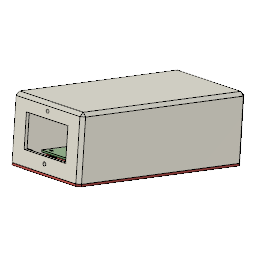
c64-psu-2018.2 v1 (Autodesk Fusion 360 design; units mm, degrees)
Autodesk Fusion 360 part; units mm, degrees
note: some values were not read from the file. Chosen so that the rebuilt part matches the saved one: which face or edge a step refers to; which pieces of a blend or face edit are solid.
sketch "PCB" plane through (0, 0, 0) normal (0, 0, 1) x (1, 0, 0)
  line L0 (0, 0) -> (117, 0)
  line L1 (117, 0) -> (117, 74)
  line L2 (117, 74) -> (0, 74)
  line L3 (0, 74) -> (0, 0)
  circle A0 centre (5, 69) radius 1.6
  circle A1 centre (5, 5) radius 1.6
  circle A2 centre (112, 69) radius 1.6
  circle A3 centre (112, 5) radius 1.6
  dimension "d1" = 74
  dimension "d2" = 117
  dimension "d5" = 3.2
  dimension "d6" = 5
  dimension "d7" = 5
  dimension "d10" = 3.2
  dimension "d11" = 5
  dimension "d12" = 5
  dimension "d13" = 3.2
  dimension "d14" = 3.2
  dimension "d15" = 5
  dimension "d16" = 5
  dimension "d17" = 5
  dimension "d18" = 5
  measures "d5" diameter of A0
  measures "d6" distance of L0.start
  measures "d7" distance of L0.start
  measures "d10" diameter of A1
  measures "d13" diameter of A2
  measures "d14" diameter of A3
extrude "Extrude6" add sketch "PCB" along normal blind 1.6 makes body 1
move_body "Move1" bodies 1 to x (1, 0, 0) y (0, 1, 0) z (0, 0, 1) at (0, 0, 7)
sketch "bottom sketch" plane through (0, 0, 0) normal (0, 0, 1) x (1, 0, 0)
  line L0 (-28, 77) -> (129, 77)
  line L1 (129, 77) -> (129, -3)
  line L2 (129, -3) -> (-28, -3)
  line L3 (-28, -3) -> (-28, 77)
  line L4 (126.2, -0.2) -> (-25.2, -0.2)
  line L5 (-25.2, -0.2) -> (-25.2, 74.2)
  line L6 (-25.2, 74.2) -> (126.2, 74.2)
  line L7 (126.2, 74.2) -> (126.2, -0.2)
  line L8 (-25.2, 74.2) -> (-16.2, 74.2)
  line L9 (-16.2, 74.2) -> (-16.2, 65.2)
  line L10 (-16.2, 65.2) -> (-25.2, 65.2)
  line L11 (-25.2, 65.2) -> (-25.2, 74.2)
  line L12 (-25.2, -0.2) -> (-16.2, -0.2)
  line L13 (-16.2, -0.2) -> (-16.2, 8.8)
  line L14 (-16.2, 8.8) -> (-25.2, 8.8)
  line L15 (-25.2, 8.8) -> (-25.2, -0.2)
  line L16 (126.2, -0.2) -> (117.2, -0.2)
  line L17 (117.2, -0.2) -> (117.2, 8.8)
  line L18 (117.2, 8.8) -> (126.2, 8.8)
  line L19 (126.2, 8.8) -> (126.2, -0.2)
  line L20 (126.2, 74.2) -> (117.2, 74.2)
  line L21 (117.2, 74.2) -> (117.2, 65.2)
  line L22 (117.2, 65.2) -> (126.2, 65.2)
  line L23 (126.2, 65.2) -> (126.2, 74.2)
  line L24 (-17.55, 69.7) -> (-19.125, 72.428)
  line L25 (-19.125, 72.428) -> (-22.275, 72.428)
  line L26 (-22.275, 72.428) -> (-23.85, 69.7)
  line L27 (-23.85, 69.7) -> (-22.275, 66.972)
  line L28 (-22.275, 66.972) -> (-19.125, 66.972)
  line L29 (-19.125, 66.972) -> (-17.55, 69.7)
  line L30 (-17.55, 4.3) -> (-19.125, 7.028)
  line L31 (-19.125, 7.028) -> (-22.275, 7.028)
  line L32 (-22.275, 7.028) -> (-23.85, 4.3)
  line L33 (-23.85, 4.3) -> (-22.275, 1.572)
  line L34 (-22.275, 1.572) -> (-19.125, 1.572)
  line L35 (-19.125, 1.572) -> (-17.55, 4.3)
  line L36 (124.85, 69.7) -> (123.275, 72.428)
  line L37 (123.275, 72.428) -> (120.125, 72.428)
  line L38 (120.125, 72.428) -> (118.55, 69.7)
  line L39 (118.55, 69.7) -> (120.125, 66.972)
  line L40 (120.125, 66.972) -> (123.275, 66.972)
  line L41 (123.275, 66.972) -> (124.85, 69.7)
  line L42 (124.85, 4.3) -> (123.275, 7.028)
  line L43 (123.275, 7.028) -> (120.125, 7.028)
  line L44 (120.125, 7.028) -> (118.55, 4.3)
  line L45 (118.55, 4.3) -> (120.125, 1.572)
  line L46 (120.125, 1.572) -> (123.275, 1.572)
  line L47 (123.275, 1.572) -> (124.85, 4.3)
  circle A0 centre (-20.7, 69.7) radius 1.6
  circle A1 centre (-20.7, 4.3) radius 1.6
  circle A2 centre (121.7, 4.3) radius 1.6
  circle A3 centre (121.7, 69.7) radius 1.6
  circle A4 centre (5, 69) radius 4
  circle A5 centre (112, 69) radius 4
  circle A6 centre (5, 5) radius 4
  circle A7 centre (112, 5) radius 4
  dimension "d22" = 3
  dimension "d23" = 3
  dimension "d24" = 28
  dimension "d25" = 12
  dimension "d60" = 2.8
  dimension "d61" = 9
  dimension "d62" = 9
  dimension "d63" = 9
  dimension "d64" = 9
  dimension "d65" = 9
  dimension "d66" = 9
  dimension "d67" = 9
  dimension "d68" = 9
  dimension "d69" = 3.15
  dimension "d70" = 4.5
  dimension "d71" = 4.5
  dimension "d72" = 3.15
  dimension "d73" = 4.5
  dimension "d74" = 4.5
  dimension "d75" = 3.15
  dimension "d76" = 4.5
  dimension "d77" = 4.5
  dimension "d78" = 3.15
  dimension "d79" = 4.5
  dimension "d80" = 4.5
  dimension "d81" = 3.2
  dimension "d82" = 3.2
  dimension "d83" = 3.2
  dimension "d84" = 3.2
  dimension "d111" = 8
  dimension "d112" = 8
  dimension "d113" = 8
  dimension "d114" = 8
  measures "d22" distance of origin
  measures "d60" distance of L2
  measures "d61" distance of origin
  measures "d63" distance of origin
  measures "d64" distance of origin
  measures "d66" distance of origin
  measures "d69" distance of origin
  measures "d73" distance of origin
  measures "d74" distance of origin
  measures "d79" distance of origin
  measures "d80" distance of origin
  measures "d81" diameter of A0
  measures "d82" diameter of A1
  measures "d83" diameter of A2
  measures "d84" diameter of A3
  measures "d111" diameter of A4
  measures "d112" diameter of A5
  measures "d113" diameter of A6
  measures "d114" diameter of A7
sketch "bounding box" plane through (0, 0, 0) normal (0, 0, 1) x (1, 0, 0)
  line L0 (-28, 77) -> (129, 77)
  line L1 (129, 77) -> (129, -3)
  line L2 (129, -3) -> (-28, -3)
  line L3 (-28, -3) -> (-28, 77)
sketch "bottom bolt recess" plane through (0, 0, 0) normal (0, 0, 1) x (1, 0, 0)
  circle A0 centre (-20.7, 69.7) radius 2.85
  circle A1 centre (-20.7, 4.3) radius 2.85
  circle A2 centre (121.7, 69.7) radius 2.85
  circle A3 centre (121.7, 4.3) radius 2.85
  dimension "d105" = 5.7
  dimension "d106" = 5.7
  dimension "d107" = 5.7
  dimension "d108" = 5.7
  measures "d105" diameter of A0
  measures "d106" diameter of A1
  measures "d107" diameter of A2
  measures "d108" diameter of A3
sketch "PCB nut recess" plane through (0, 0, 0) normal (0, 0, 1) x (1, 0, 0)
  line L0 (6.575, 66.272) -> (8.15, 69)
  line L1 (8.15, 69) -> (6.575, 71.728)
  line L2 (6.575, 71.728) -> (3.425, 71.728)
  line L3 (3.425, 71.728) -> (1.85, 69)
  line L4 (1.85, 69) -> (3.425, 66.272)
  line L5 (3.425, 66.272) -> (6.575, 66.272)
  line L6 (8.15, 5) -> (6.575, 7.728)
  line L7 (6.575, 7.728) -> (3.425, 7.728)
  line L8 (3.425, 7.728) -> (1.85, 5)
  line L9 (1.85, 5) -> (3.425, 2.272)
  line L10 (3.425, 2.272) -> (6.575, 2.272)
  line L11 (6.575, 2.272) -> (8.15, 5)
  line L12 (110.425, 66.272) -> (113.575, 66.272)
  line L13 (113.575, 66.272) -> (115.15, 69)
  line L14 (115.15, 69) -> (113.575, 71.728)
  line L15 (113.575, 71.728) -> (110.425, 71.728)
  line L16 (110.425, 71.728) -> (108.85, 69)
  line L17 (108.85, 69) -> (110.425, 66.272)
  line L18 (108.3627, 5) -> (110.1813, 1.85)
  line L19 (110.1813, 1.85) -> (113.8187, 1.85)
  line L20 (113.8187, 1.85) -> (115.6373, 5)
  line L21 (115.6373, 5) -> (113.8187, 8.15)
  line L22 (113.8187, 8.15) -> (110.1813, 8.15)
  line L23 (110.1813, 8.15) -> (108.3627, 5)
  dimension "d118" = 3.15
  dimension "d119" = 3.15
  dimension "d120" = 3.15
  dimension "d121" = 3.15
  measures "d121" distance of L23
sketch "PCB holes" plane through (0, 0, 0) normal (0, 0, 1) x (1, 0, 0)
  circle A0 centre (5, 69) radius 1.6
  circle A1 centre (5, 5) radius 1.6
  circle A2 centre (112, 69) radius 1.6
  circle A3 centre (112, 5) radius 1.6
  dimension "d124" = 3.2
  dimension "d125" = 3.2
  dimension "d126" = 3.2
  dimension "d127" = 3.2
  measures "d124" diameter of A0
  measures "d125" diameter of A1
  measures "d126" diameter of A2
  measures "d127" diameter of A3
extrude "Extrude9" add sketch "bottom sketch" along normal blind 2 separate body contours L0 L1 L2 L3 makes body 2
extrude "Extrude10" add sketch "bottom sketch" along normal blind 4 contours L4 L5 L6 L7 L9 L10 L13 L14 L17 L18 L21 L22 | A4 | A5 | A6 | A7 bodies 2
extrude "Extrude11" add sketch "bottom sketch" along normal blind 6 contours L4 L7 L16 L17 L18 L19 | L4 L5 L12 L13 L14 L15 | L6 L7 L20 L21 L22 L23 | L5 L6 L8 L9 L10 L11 bodies 2
extrude "Extrude12" add sketch "bottom sketch" along normal blind 6 contours L24 L25 L26 L27 L28 L29 | L30 L31 L32 L33 L34 L35 | L36 L37 L38 L39 L40 L41 | L42 L43 L44 L45 L46 L47 bodies 2
extrude "Extrude15" add sketch "bottom sketch" along normal blind 7 contours A4 | A5 | A6 | A7 bodies 2
extrude "Extrude14" cut sketch "bottom bolt recess" along normal blind 3.5 bodies 2
extrude "Extrude17" cut sketch "PCB holes" along normal through all bodies 2
extrude "Extrude16" cut sketch "PCB nut recess" along normal blind 4 bodies 2
chamfer "Chamfer4" distance 3 angle 45 4 edges at (-28, -3, 1) (129, -3, 1) (129, 77, 1) (-28, 77, 1) on bodies 2
chamfer "Chamfer5" distance 2 angle 45 4 edges at (126.2, -0.2, 4) (126.2, 74.2, 4) (-25.2, 74.2, 4) (-25.2, -0.2, 4) on bodies 2
move_face "OffsetFaces1" offset -0.2 4 faces at (126.2, 69.8667, 4) (-20.8667, 74.2, 4) (121.8667, -0.2, 4) (-25.2, 69.8667, 4) on bodies 2
ref_plane "WorkPlane3" through (5, 69, 7) normal (0, 0, 1) x (1, 0, 0)
ref_plane "WorkPlane4" through (50.5, 37, 2) normal (0, 0, 1) x (1, 0, 0)
ref_plane "WorkPlane5" through (-20.7, 4.3, 6) normal (0, 0, 1) x (1, 0, 0)
copy_body "Body->Comp1" bodies 2 removing the originals makes body 3 in component "c64-psu-bottom-v2018.2"
extrude "Extrude18" add sketch "bottom sketch" along normal blind 52 from surface at 2 separate body contours L0 L1 L2 L3 makes body 4
extrude "Extrude19" add sketch "bottom sketch" along normal blind 6 from surface at 6 contours L4 L7 L16 L17 L18 L19 | L4 L5 L12 L13 L14 L15 | L6 L7 L20 L21 L22 L23 | L5 L6 L8 L9 L10 L11 | L24 L25 L26 L27 L28 L29 | L30 L31 L32 L33 L34 L35 | L36 L37 L38 L39 L40 L41 | L42 L43 L44 L45 L46 L47 bodies 4
extrude "Extrude20" cut sketch "bottom sketch" along normal blind 4 from surface at 8 contours L24 L25 L26 L27 L28 L29 | L30 L31 L32 L33 L34 L35 | L36 L37 L38 L39 L40 L41 | L42 L43 L44 L45 L46 L47 bodies 4
extrude "Extrude21" add sketch "bounding box" along normal blind 2 from surface at 54 bodies 4
sketch "high voltage holes" plane through (0, 0, 0) normal (1, 0, 0) x (0, 1, 0)
  line L0 (61.05, 14.75) -> (12.95, 14.75)
  line L1 (12.95, 14.75) -> (12.95, 43.25)
  line L2 (12.95, 43.25) -> (61.05, 43.25)
  line L3 (61.05, 43.25) -> (61.05, 14.75)
  circle A0 centre (37, 49) radius 1.6
  circle A1 centre (37, 9) radius 1.6
  line L4 (37, -11.0746) -> (37, 71.9112) construction
  line L5 (81.9395, 29) -> (-15, 29) construction
  line L6 (77, 2) -> (77, 56)
  line L7 (49, 9) -> (21, 9) construction
  line L8 (26, 49) -> (52, 49) construction
  line L9 (32.5, 4.5) -> (41.5, 4.5)
  line L10 (41.5, 4.5) -> (41.5, 13.5)
  line L11 (41.5, 13.5) -> (32.5, 13.5)
  line L12 (32.5, 13.5) -> (32.5, 4.5)
  line L13 (34.272, 7.425) -> (37, 5.85)
  line L14 (37, 5.85) -> (39.728, 7.425)
  line L15 (39.728, 7.425) -> (39.728, 10.575)
  line L16 (39.728, 10.575) -> (37, 12.15)
  line L17 (37, 12.15) -> (34.272, 10.575)
  line L18 (34.272, 10.575) -> (34.272, 7.425)
  line L19 (41.5, 44.5) -> (32.5, 44.5)
  line L20 (32.5, 44.5) -> (32.5, 53.5)
  line L21 (32.5, 53.5) -> (41.5, 53.5)
  line L22 (41.5, 53.5) -> (41.5, 44.5)
  line L23 (39.728, 50.575) -> (37, 52.15)
  line L24 (37, 52.15) -> (34.272, 50.575)
  line L25 (34.272, 50.575) -> (34.272, 47.425)
  line L26 (34.272, 47.425) -> (37, 45.85)
  line L27 (37, 45.85) -> (39.728, 47.425)
  line L28 (39.728, 47.425) -> (39.728, 50.575)
  dimension "d143" = 48.1
  dimension "d144" = 28.5
  dimension "d145" = 3.2
  dimension "d146" = 3.2
  dimension "d147" = 40
  dimension "d148" = 9
  dimension "d149" = 9
  dimension "d150" = 9
  dimension "d151" = 3.15
  dimension "d152" = 9
  dimension "d153" = 9
  dimension "d154" = 3.15
  measures "d143" distance of origin
  measures "d145" diameter of A0
  measures "d146" diameter of A1
  measures "d147" distance of origin
  measures "d148" distance of origin
extrude "Extrude22" add sketch "high voltage holes" along normal blind 5 from surface at -25.2 contours L9 L10 L11 L12 | L13 L14 L15 L16 L17 L18 | L19 L20 L21 L22 | L23 L24 L25 L26 L27 L28 bodies 4
extrude "Extrude23" cut sketch "high voltage holes" against normal blind 4 from surface at -20.2 contours L13 L14 L15 L16 L17 L18 | L23 L24 L25 L26 L27 L28 bodies 4
extrude "Extrude24" cut sketch "high voltage holes" along normal blind 10 from surface at -28 contours L0 L1 L2 L3 | A0 | A1 bodies 4
sketch "Sketch12" plane through (0, 0, 0) normal (1, 0, 0) x (0, 1, 0)
  line L0 (37, -11.0746) -> (37, 71.9112) construction
  circle A0 centre (37, 17) radius 6.3
  dimension "d166" = 12.6
  dimension "d167" = 17
  measures "d166" diameter of A0
  measures "d167" distance of origin
extrude "Extrude25" cut sketch "Sketch12" against normal blind 20 from surface at 129 bodies 4
chamfer "Chamfer2" distance 3 angle 45 8 edges at (129, 37, 56) (50.5, 77, 56) (-28, 37, 56) (50.5, -3, 56) (-28, 77, 29) (-28, -3, 29) (129, -3, 29) (129, 77, 29) on bodies 4
chamfer "Chamfer3" distance 2 angle 45 13 edges at (126.2, -0.2, 4) (126.2, 74.2, 4) (126.2, -0.2, 33) (126.2, 74.2, 33) (126.2, 37, 54) (50.5, -0.2, 54) (-25.2, -0.2, 33) (-25.2, -0.2, 4) (-25.2, 74.2, 4) (-25.2, 74.2, 33) (-25.2, 37, 54) (-25.2, 37, 53.5) (50.5, 74.2, 54) on bodies 4
copy_body "Body->Comp2" bodies 4 removing the originals makes body 5 in component "c64-psu-top-v2018.2"
component "c64-psu-bottom-v2018.2" placed x (1, 0, 0) y (0, 1, 0) z (0, 0, 1) at (0, 0, 0)
component "c64-psu-top-v2018.2" placed x (1, 0, 0) y (0, 1, 0) z (0, 0, 1) at (0, 0, 0)
named bodies: "PCB"
